Autodesk Inventor part; units mm, degrees
(part 2 of 2)
fillet "Fillet1" radius 4 4 edges at (-72.1915, 62.8097, 3.5) (-88.7804, -31.274, 3.5) (198.4911, 62.8097, 3.5) (215.0786, -31.2745, 3.5)
fillet "Fillet2" radius 4 10 edges at (-71.4063, 61.8738, 7) (-80.4411, 16.0224, 7) (-87.4817, -30.3953, 7) (-30.1108, -43.5751, 7) (197.7059, 61.8738, 7) (206.74, 16.0221, 7) (213.7798, -30.3958, 7) (156.4089, -43.5753, 7) (63.1498, 62.8097, 7) (63.149, -55.0813, 7)
fillet "Fillet3" radius 1 28 edges at (-62.9014, 53.3064, 4.5) (-24.9574, 49.6622, 4.5) (-5.3778, 51.287, 4.5) (14.5153, 47.7794, 4.5) (32.1848, 38.5712, 4.5) (50.0279, 30.3479, 4.5) (-76.3066, -22.7207, 4.5) (-37.702, -29.5275, 4.5) (-18.5275, -29.8623, 4.5) (36.6224, -45.6793, 4.5) (16.7292, -42.1717, 4.5) (-1.1139, -33.9484, 4.5) (70.4439, -46.0074, 4.5) (89.6759, -45.6797, 4.5) (109.5691, -42.1725, 4.5) (127.4123, -33.9494, 4.5) (144.826, -29.8637, 4.5) (164.0005, -29.5291, 4.5) (202.6052, -22.723, 4.5) (189.2012, 53.3044, 4.5) (151.2572, 49.6608, 4.5) (131.6776, 51.2859, 4.5) (111.7844, 47.7786, 4.5) (94.1148, 38.5707, 4.5) (76.2716, 30.3477, 4.5) (63.6397, -7.4141, 4.5) (62.6592, -7.4141, 4.5) (55.8544, -46.0073, 4.5)
equation "\"d9\" = d8"
equation "\"d10\" = d8"
equation "\"d11\" = d8"
equation "\"d12\" = d8"
equation "\"d13\" = d8"
equation "\"d14\" = d8"
equation "\"d15\" = d8"
equation "\"d16\" = d8"
equation "\"d17\" = d8"
equation "\"d18\" = d8"
equation "\"d19\" = d8"
equation "\"d20\" = d8"
equation "\"d21\" = d8"
equation "\"d22\" = d8"
equation "\"d23\" = d8"
equation "\"d24\" = d8"
equation "\"d25\" = d8"
equation "\"d26\" = d8"
equation "\"d27\" = d8"
equation "\"d28\" = d8"
equation "\"d32\" = d8"
equation "\"d33\" = d8"
equation "\"d34\" = d8"
equation "\"d1\" = d0"
equation "\"d3\" = d0"
equation "\"d4\" = d0"
equation "\"d5\" = d0"
equation "\"d0\" = 9"
body "Solid1"
